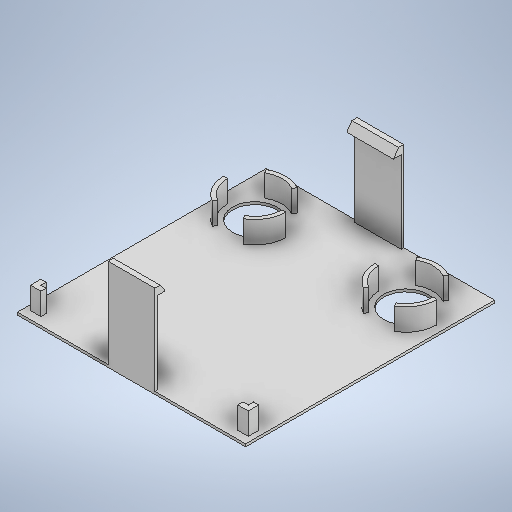
# Autodesk Inventor part: case_v1
Saved by Autodesk Inventor 2025 (Build 290162000, 162)
## iProperties
Created: 2025-03-20
Part Number: case_v1
Material: Generic
Document SubType Name: Modeling
Designer: ethan
Density: 1 g/cm^3
Appearance: Default
Author: ethan
Autodesk Inventor part; units mm, degrees
ref_plane "YZ Plane" through (0, 0, 0) normal (1, 0, 0) x (0, 1, 0)
ref_plane "XZ Plane" through (0, 0, 0) normal (0, 1, 0) x (-1, 0, 0)
ref_plane "XY Plane" through (0, 0, 0) normal (0, 0, 1) x (1, 0, 0)
sketch "Sketch1" plane through (0, 0, 0) normal (0, 1, 0) x (-1, 0, 0)
  line L0 (0, 0) -> (-88, 0)
  line L1 (-88, 0) -> (-88, -94)
  line L2 (-88, -94) -> (0, -94)
  line L3 (0, -94) -> (0, 0)
  line L4 (0, -94) -> (0, -75.65)
  line L5 (0, -94) -> (-14.85, -94)
  circle A0 centre (-14.85, -75.65) radius 8.5
  line L6 (-44, -88.9444) -> (-44, -54.2543) construction
  circle A1 centre (-73.15, -75.65) radius 8.5
  dimension "d0" = 88
  dimension "d1" = 94
  dimension "d2" = 18.35
  dimension "d3" = 14.85
  dimension "d4" = 17
  constraints: 14 end point, 2 centre point, 2 parallel, 2 point on line, 1 horizontal, 1 perpendicular, 1 symmetric about line, 1 vertical, 1 other
  measures "d0" distance of L2.end L1.end
  measures "d1" distance of L1.end L0.end
  measures "d2" distance of L2.end L4.end
  measures "d3" distance of L2.end L5.end
  measures "d4" diameter of A0
extrude "Extrusion1" add sketch "Sketch1" along normal blind 1
sketch "Sketch2" plane through (0, 1, 0) normal (0, 1, 0) x (1, 0, 0)
  line L0 (88, 94) -> (0, 94) construction
  line L1 (0, 94) -> (0, 0) construction
  line L2 (0, 0) -> (88, 0) construction
  line L3 (88, 0) -> (88, 94) construction
  circle A0 centre (73.15, 75.65) radius 8.5 construction
  circle A1 centre (14.85, 75.65) radius 8.5 construction
  line L4 (0, 94) -> (88, 94) construction
  line L5 (88, 94) -> (88, 95) construction
  line L6 (88, 95) -> (0, 95) construction
  line L7 (0, 95) -> (0, 94) construction
  line L8 (0, 0) -> (88, 0) construction
  line L9 (88, 0) -> (88, -1) construction
  line L10 (88, -1) -> (0, -1) construction
  line L11 (0, -1) -> (0, 0) construction
  line L12 (88, 95) -> (0, 95)
  line L13 (0, 95) -> (0, 94)
  line L14 (0, 94) -> (88, 94)
  line L15 (88, 94) -> (88, 95)
  line L16 (0, 0) -> (88, 0)
  line L17 (88, 0) -> (88, -1)
  line L18 (88, -1) -> (0, -1)
  line L19 (0, -1) -> (0, 0)
  dimension "d7" = 1
  dimension "d8" = 1
  constraints: 32 end point, 8 parallel, 4 horizontal, 4 perpendicular, 1 point on line
  measures "d7" distance of L5.end L4.end
  measures "d8" distance of L8.end L9.end
extrude "Extrusion2" add sketch "Sketch2" against normal blind 1
sketch "Sketch3" plane through (0, 1, 0) normal (0, 1, 0) x (1, 0, 0)
  line L0 (0, 95) -> (0, -1) construction
  line L1 (0, -1) -> (88, -1) construction
  line L2 (88, -1) -> (88, 95) construction
  line L3 (88, 95) -> (0, 95) construction
  circle A0 centre (73.15, 75.65) radius 8.5 construction
  circle A1 centre (14.85, 75.65) radius 8.5 construction
  line L4 (0, 0) -> (4, 0) construction
  line L5 (4, 0) -> (4, 4) construction
  line L6 (4, 4) -> (0, 4) construction
  line L7 (0, 4) -> (0, 0) construction
  line L8 (88, 0) -> (84, 0) construction
  line L9 (84, 0) -> (84, 4) construction
  line L10 (84, 4) -> (88, 4) construction
  line L11 (88, 4) -> (88, 0) construction
  line L12 (4, 4) -> (2, 4) construction
  line L13 (2, 4) -> (2, 2) construction
  line L14 (2, 2) -> (4, 2) construction
  line L15 (4, 2) -> (4, 4) construction
  line L16 (2, 2) -> (6, 2)
  line L17 (6, 2) -> (6, 4)
  line L18 (6, 4) -> (2, 4)
  line L19 (2, 4) -> (2, 2)
  line L20 (2, 2) -> (4, 2)
  line L21 (4, 2) -> (4, 6)
  line L22 (4, 6) -> (2, 6)
  line L23 (2, 6) -> (2, 2)
  line L24 (86, 2) -> (82, 2)
  line L25 (82, 2) -> (82, 4)
  line L26 (82, 4) -> (86, 4)
  line L27 (86, 4) -> (86, 2)
  line L28 (86, 2) -> (84, 2)
  line L29 (84, 2) -> (84, 6)
  line L30 (84, 6) -> (86, 6)
  line L31 (86, 6) -> (86, 2)
  line L32 (44, 4.3599) -> (37, 4.3599) construction
  line L33 (88, -1) -> (0, -1) construction
  line L34 (37, -1) -> (51, -1) construction
  line L35 (51, -1) -> (51, 0) construction
  line L36 (51, 0) -> (37, 0) construction
  line L37 (37, 0) -> (37, -1) construction
  line L38 (37, -1) -> (51, -1)
  line L39 (51, -1) -> (51, 0)
  line L40 (51, 0) -> (37, 0)
  line L41 (37, 0) -> (37, -1)
  line L42 (0, 95) -> (88, 95) projected
  line L43 (37, 95) -> (51, 95)
  line L44 (51, 95) -> (51, 94)
  line L45 (51, 94) -> (37, 94)
  line L46 (37, 94) -> (37, 95)
  circle A2 centre (14.85, 75.65) radius 10.5
  circle A3 centre (14.85, 75.65) radius 12
  line L47 (14.85, 75.65) -> (26.85, 75.65) construction
  line L48 (14.85, 75.65) -> (20.85, 86.0423) construction
  line L49 (14.85, 75.65) -> (8.85, 86.0423) construction
  line L50 (14.85, 75.65) -> (2.85, 75.65) construction
  line L51 (14.85, 75.65) -> (8.85, 65.2577) construction
  line L52 (14.85, 75.65) -> (20.85, 65.2577) construction
  line L53 (9.6, 84.7433) -> (8.85, 86.0423) construction
  line L54 (9.6, 84.7433) -> (8.85, 86.0423)
  line L55 (20.85, 86.0423) -> (20.1, 84.7433)
  line L56 (25.35, 75.65) -> (26.85, 75.65)
  line L57 (20.85, 65.2577) -> (20.1, 66.5567)
  line L58 (9.6, 66.5567) -> (8.85, 65.2577)
  line L59 (4.35, 75.65) -> (2.85, 75.65)
  line L60 (44, 84.7433) -> (44, 74.6259) construction
  circle A4 centre (73.15, 75.65) radius 8.5 construction
  circle A5 centre (73.15, 75.65) radius 10.5
  circle A6 centre (73.15, 75.65) radius 12
  line L61 (73.15, 75.65) -> (61.15, 75.65) construction
  line L62 (73.15, 75.65) -> (67.15, 86.0423) construction
  line L63 (73.15, 75.65) -> (79.15, 86.0423) construction
  line L64 (73.15, 75.65) -> (85.15, 75.65) construction
  line L65 (73.15, 75.65) -> (79.15, 65.2577) construction
  line L66 (73.15, 75.65) -> (67.15, 65.2577) construction
  line L67 (78.4, 84.7433) -> (79.15, 86.0423) construction
  line L68 (78.4, 84.7433) -> (79.15, 86.0423)
  line L69 (67.15, 86.0423) -> (67.9, 84.7433)
  line L70 (62.65, 75.65) -> (61.15, 75.65)
  line L71 (67.15, 65.2577) -> (67.9, 66.5567)
  line L72 (78.4, 66.5567) -> (79.15, 65.2577)
  line L73 (83.65, 75.65) -> (85.15, 75.65)
  point P0 (84, 4)
  dimension "d11" = 4
  dimension "d12" = 4
  dimension "d13" = 4
  dimension "d14" = 4
  dimension "d15" = 2
  dimension "d16" = 2
  dimension "d17" = 4
  dimension "d18" = 4
  dimension "d19" = 4
  dimension "d20" = 2
  dimension "d21" = 4
  dimension "d22" = 7
  dimension "d23" = 14
  dimension "d24" = 14
  dimension "d25" = 1
  dimension "d26" = 2
  dimension "d27" = 1.5
  dimension "d30" = 360
  constraints: 136 end point, 20 parallel, 20 point on line, 19 symmetric about line, 16 point on circle, 10 perpendicular, 9 horizontal, 5 centre point, 5 collinear, 2 coincident, 1 vertical, 20 other
  measures "d11" distance of L6.end L5.end
  measures "d12" distance of L5.end L4.end
  measures "d13" distance of L9.end L10.end
  measures "d14" distance of L8.end L9.end
  measures "d15" distance of L14.end L13.end
  measures "d16" distance of L13.end L12.end
  measures "d17" distance of L18.end L17.end
  measures "d18" distance of L21.end L20.end
  measures "d19" distance of L25.end L26.end
  measures "d20" distance of L29.end L30.end
  measures "d21" distance of L28.end L29.end
  measures "d22" distance of L32.start L32.end
  measures "d23" distance of L34.start L34.end
  measures "d24" distance of L43.start L43.end
  measures "d25" distance of L43.end L44.end
  measures "d26" radial gap between concentric circles of A1 A2
  measures "d27" radial gap between concentric circles of A2 A3
extrude "Extrusion3" add sketch "Sketch3" along normal blind 8.5 contours L19 L18 L21 L16 | L21 L18 L17 L16 | L23 L22 L21 L18 | L24 L29 L26 L27 | L24 L25 L26 L29 | L26 L29 L30 L31 | L56 A3 L57 A2 | A2 L54 A3 L55 | L58 A3 L59 A2 | L73 A6 L72 A5 | A5 L69 A6 L68 | L71 A6 L70 A5
sketch "Sketch4" plane through (0, 1, 0) normal (0, 1, 0) x (1, 0, 0)
  line L0 (2.85, 75.65) -> (4.35, 75.65) construction
  arc A0 (4.35, 75.65) -> (9.6, 66.5567) centre (14.85, 75.65) ccw construction
  line L1 (9.6, 66.5567) -> (8.85, 65.2577) construction
  arc A1 (2.85, 75.65) -> (8.85, 65.2577) centre (14.85, 75.65) ccw construction
  line L2 (84, 6) -> (86, 6) construction
  line L3 (86, 6) -> (86, 2) construction
  line L4 (86, 2) -> (82, 2) construction
  line L5 (82, 2) -> (82, 4) construction
  line L6 (82, 4) -> (84, 4) construction
  line L7 (84, 4) -> (84, 6) construction
  arc A2 (62.65, 75.65) -> (67.9, 66.5567) centre (73.15, 75.65) ccw construction
  line L8 (67.9, 66.5567) -> (67.15, 65.2577) construction
  arc A3 (61.15, 75.65) -> (67.15, 65.2577) centre (73.15, 75.65) ccw construction
  line L9 (61.15, 75.65) -> (62.65, 75.65) construction
  line L10 (25.35, 75.65) -> (26.85, 75.65) construction
  arc A4 (20.85, 65.2577) -> (26.85, 75.65) centre (14.85, 75.65) ccw construction
  line L11 (20.85, 65.2577) -> (20.1, 66.5567) construction
  arc A5 (20.1, 66.5567) -> (25.35, 75.65) centre (14.85, 75.65) ccw construction
  arc A6 (78.4, 84.7433) -> (67.9, 84.7433) centre (73.15, 75.65) ccw construction
  line L12 (67.9, 84.7433) -> (67.15, 86.0423) construction
  arc A7 (79.15, 86.0423) -> (67.15, 86.0423) centre (73.15, 75.65) ccw construction
  line L13 (79.15, 86.0423) -> (78.4, 84.7433) construction
  line L14 (2, 6) -> (4, 6) construction
  line L15 (4, 6) -> (4, 4) construction
  line L16 (4, 4) -> (6, 4) construction
  line L17 (6, 4) -> (6, 2) construction
  line L18 (6, 2) -> (2, 2) construction
  line L19 (2, 2) -> (2, 6) construction
  line L20 (83.65, 75.65) -> (85.15, 75.65) construction
  arc A8 (79.15, 65.2577) -> (85.15, 75.65) centre (73.15, 75.65) ccw construction
  line L21 (79.15, 65.2577) -> (78.4, 66.5567) construction
  arc A9 (78.4, 66.5567) -> (83.65, 75.65) centre (73.15, 75.65) ccw construction
  line L22 (20.85, 86.0423) -> (20.1, 84.7433) construction
  arc A10 (20.1, 84.7433) -> (9.6, 84.7433) centre (14.85, 75.65) ccw construction
  line L23 (9.6, 84.7433) -> (8.85, 86.0423) construction
  arc A11 (20.85, 86.0423) -> (8.85, 86.0423) centre (14.85, 75.65) ccw construction
  line L24 (0, 95) -> (0, -1) construction
  line L25 (0, -1) -> (88, -1) construction
  line L26 (88, -1) -> (88, 95) construction
  line L27 (88, 95) -> (0, 95) construction
  circle A12 centre (73.15, 75.65) radius 8.5 construction
  circle A13 centre (14.85, 75.65) radius 8.5 construction
  line L28 (44, 63.0064) -> (44, 95) construction
  line L29 (88, 95) -> (0, 95) construction
  line L30 (44, 95) -> (53, 95) construction
  line L31 (53, 95) -> (35, 95) construction
  line L32 (35, 95) -> (53, 95) construction
  line L33 (53, 95) -> (53, 94) construction
  line L34 (53, 94) -> (35, 94) construction
  line L35 (35, 94) -> (35, 95) construction
  line L36 (35, 95) -> (53, 95)
  line L37 (53, 95) -> (53, 94)
  line L38 (53, 94) -> (35, 94)
  line L39 (35, 94) -> (35, 95)
  line L40 (34.0602, 47) -> (52.5165, 47)
  line L41 (44, -1) -> (53, -1) construction
  line L42 (53, -1) -> (35, -1) construction
  line L43 (35, -1) -> (53, -1) construction
  line L44 (53, -1) -> (53, 0) construction
  line L45 (53, 0) -> (35, 0) construction
  line L46 (35, 0) -> (35, -1) construction
  line L47 (35, -1) -> (53, -1)
  line L48 (53, -1) -> (53, 0)
  line L49 (53, 0) -> (35, 0)
  line L50 (35, 0) -> (35, -1)
  point P0 (0, 0)
  dimension "d34" = 9
  dimension "d35" = 18
  dimension "d36" = 1
  constraints: 44 end point, 7 symmetric about line, 4 parallel, 2 collinear, 2 perpendicular, 2 point on line, 1 horizontal, 1 midpoint
  measures "d34" distance of L28.end L30.end
  measures "d35" distance of L30.end L31.end
  measures "d36" distance of L30.end L33.end
extrude "Extrusion4" add sketch "Sketch4" along normal blind 34.5
sketch "Sketch5" plane through (53, 1, 1) normal (1, 0, 0) x (0, 0, -1)
  line L0 (1, 0) -> (0, 0) construction
  line L1 (1, 0) -> (1, 34.5) construction
  line L2 (0, 34.5) -> (1, 34.5) construction
  line L3 (0, 0) -> (0, 34.5) construction
  line L4 (96, -1) -> (0, -1) construction
  line L5 (96, 0) -> (96, -1) construction
  line L6 (0, 0) -> (96, 0) construction
  line L7 (0, 0) -> (0, -1) construction
  line L8 (96, 0) -> (96, 34.5) construction
  line L9 (96, 0) -> (95, 0) construction
  line L10 (96, 0) -> (96, 34.5) construction
  line L11 (95, 34.5) -> (96, 34.5) construction
  line L12 (95, 0) -> (95, 34.5) construction
  line L13 (0, 34.5) -> (0, 31.6) construction
  line L14 (1, 31.6) -> (4, 31.6) construction
  line L15 (1, 34.5) -> (2, 34.5) construction
  line L16 (2, 34.5) -> (4, 31.6) construction
  line L17 (0, 34.5) -> (2, 34.5)
  line L18 (4, 31.6) -> (2, 34.5)
  line L19 (4, 31.6) -> (0, 31.6)
  line L20 (0, 31.6) -> (0, 34.5)
  line L21 (0, -1) -> (96, -1) projected
  line L22 (48, -1) -> (48, 2.5166)
  line L23 (95, 0) -> (95, 34.5) construction
  line L24 (96, 34.5) -> (95, 34.5) construction
  line L25 (96, 0) -> (96, 34.5) construction
  line L26 (96, 34.5) -> (96, 31.6) construction
  line L27 (95, 31.6) -> (92, 31.6) construction
  line L28 (95, 34.5) -> (94, 34.5) construction
  line L29 (94, 34.5) -> (92, 31.6) construction
  line L30 (96, 34.5) -> (94, 34.5)
  line L31 (92, 31.6) -> (94, 34.5)
  line L32 (92, 31.6) -> (96, 31.6)
  line L33 (96, 31.6) -> (96, 34.5)
  point P0 (1, -1)
  dimension "d39" = 2.9
  dimension "d40" = 3
  dimension "d41" = 1
  constraints: 40 end point, 5 symmetric about line, 4 point on line, 3 collinear, 2 perpendicular, 1 horizontal, 1 midpoint, 1 vertical
  measures "d39" distance of L2.start L13.end
  measures "d40" distance of L14.start L14.end
  measures "d41" distance of L1.end L15.end
extrude "Extrusion5" add sketch "Sketch5" against normal up to surface (18 mm away)
equation "\"d42\" = d40"
body "Solid1"
